Autodesk Inventor part; units mm, degrees
(part 4 of 4)
  line L354 (-31.6525, 241.1962) -> (-31.6525, 254.1962)
  line L355 (-17.6525, 241.1962) -> (-17.6525, 254.1962)
  line L356 (-31.1525, 240.6962) -> (-18.1525, 240.6962)
  line L357 (-31.1525, 254.6962) -> (-18.1525, 254.6962)
  arc A352 (-31.6525, 241.1962) -> (-31.1525, 240.6962) centre (-31.1525, 241.1962) ccw
  arc A353 (-31.1525, 254.6962) -> (-31.6525, 254.1962) centre (-31.1525, 254.1962) ccw
  arc A354 (-18.1525, 240.6962) -> (-17.6525, 241.1962) centre (-18.1525, 241.1962) ccw
  arc A355 (-17.6525, 254.1962) -> (-18.1525, 254.6962) centre (-18.1525, 254.1962) ccw
  line L358 (-31.6525, 265.0087) -> (-31.6525, 278.0087)
  line L359 (-17.6525, 265.0087) -> (-17.6525, 278.0087)
  line L360 (-31.1525, 264.5087) -> (-18.1525, 264.5087)
  line L361 (-31.1525, 278.5087) -> (-18.1525, 278.5087)
  arc A356 (-31.6525, 265.0087) -> (-31.1525, 264.5087) centre (-31.1525, 265.0087) ccw
  arc A357 (-31.1525, 278.5087) -> (-31.6525, 278.0087) centre (-31.1525, 278.0087) ccw
  arc A358 (-18.1525, 264.5087) -> (-17.6525, 265.0087) centre (-18.1525, 265.0087) ccw
  arc A359 (-17.6525, 278.0087) -> (-18.1525, 278.5087) centre (-18.1525, 278.0087) ccw
  line L362 (-31.6525, 288.8212) -> (-31.6525, 301.8212)
  line L363 (-17.6525, 288.8212) -> (-17.6525, 301.8212)
  line L364 (-31.1525, 288.3212) -> (-18.1525, 288.3212)
  line L365 (-31.1525, 302.3212) -> (-18.1525, 302.3212)
  arc A360 (-31.6525, 288.8212) -> (-31.1525, 288.3212) centre (-31.1525, 288.8212) ccw
  arc A361 (-31.1525, 302.3212) -> (-31.6525, 301.8212) centre (-31.1525, 301.8212) ccw
  arc A362 (-18.1525, 288.3212) -> (-17.6525, 288.8212) centre (-18.1525, 288.8212) ccw
  arc A363 (-17.6525, 301.8212) -> (-18.1525, 302.3212) centre (-18.1525, 301.8212) ccw
  line L366 (-31.6525, 315.015) -> (-31.6525, 328.015)
  line L367 (-17.6525, 315.015) -> (-17.6525, 328.015)
  line L368 (-31.1525, 314.515) -> (-18.1525, 314.515)
  line L369 (-31.1525, 328.515) -> (-18.1525, 328.515)
  arc A364 (-31.6525, 315.015) -> (-31.1525, 314.515) centre (-31.1525, 315.015) ccw
  arc A365 (-31.1525, 328.515) -> (-31.6525, 328.015) centre (-31.1525, 328.015) ccw
  arc A366 (-18.1525, 314.515) -> (-17.6525, 315.015) centre (-18.1525, 315.015) ccw
  arc A367 (-17.6525, 328.015) -> (-18.1525, 328.515) centre (-18.1525, 328.015) ccw
  line L370 (-31.6525, 334.065) -> (-31.6525, 347.065)
  line L371 (-17.6525, 334.065) -> (-17.6525, 347.065)
  line L372 (-31.1525, 333.565) -> (-18.1525, 333.565)
  line L373 (-31.1525, 347.565) -> (-18.1525, 347.565)
  arc A368 (-31.6525, 334.065) -> (-31.1525, 333.565) centre (-31.1525, 334.065) ccw
  arc A369 (-31.1525, 347.565) -> (-31.6525, 347.065) centre (-31.1525, 347.065) ccw
  arc A370 (-18.1525, 333.565) -> (-17.6525, 334.065) centre (-18.1525, 334.065) ccw
  arc A371 (-17.6525, 347.065) -> (-18.1525, 347.565) centre (-18.1525, 347.065) ccw
  line L374 (-31.6525, 353.115) -> (-31.6525, 366.115)
  line L375 (-17.6525, 353.115) -> (-17.6525, 366.115)
  line L376 (-31.1525, 352.615) -> (-18.1525, 352.615)
  line L377 (-31.1525, 366.615) -> (-18.1525, 366.615)
  arc A372 (-31.6525, 353.115) -> (-31.1525, 352.615) centre (-31.1525, 353.115) ccw
  arc A373 (-31.1525, 366.615) -> (-31.6525, 366.115) centre (-31.1525, 366.115) ccw
  arc A374 (-18.1525, 352.615) -> (-17.6525, 353.115) centre (-18.1525, 353.115) ccw
  arc A375 (-17.6525, 366.115) -> (-18.1525, 366.615) centre (-18.1525, 366.115) ccw
  line L378 (-15.1275, 21.4775) -> (-15.1275, 369.14)
  line L379 (-134.19, 21.4775) -> (-134.19, 369.14)
  line L380 (-15.1275, 21.4775) -> (-134.19, 21.4775)
  line L381 (-15.1275, 369.14) -> (-134.19, 369.14)
  point P0 (0, 0)
  point P1 (-118.165, 271.6525)
  point P2 (-117.665, 272.1525)
  point P3 (-117.665, 285.1525)
  point P4 (-118.165, 285.6525)
  point P5 (-131.665, 285.1525)
  point P6 (-131.665, 272.1525)
  point P7 (-107.8525, 315.015)
  point P8 (-107.3525, 314.515)
  point P9 (-94.3525, 314.515)
  point P10 (-93.8525, 315.015)
  point P11 (-93.8525, 328.015)
  point P12 (-94.3525, 328.515)
  point P13 (-107.8525, 328.015)
  point P14 (-93.8525, 334.065)
  point P15 (-93.8525, 347.065)
  point P16 (-94.3525, 347.565)
  point P17 (-107.3525, 347.565)
  point P18 (-107.8525, 347.065)
  point P19 (-107.8525, 334.065)
  point P20 (-107.3525, 352.615)
  point P21 (-94.3525, 352.615)
  point P22 (-93.8525, 353.115)
  point P23 (-94.3525, 366.615)
  point P24 (-107.3525, 366.615)
  point P25 (-107.8525, 366.115)
  point P26 (-107.8525, 353.115)
  point P27 (-31.1525, 314.515)
  point P28 (-18.1525, 314.515)
  point P29 (-17.6525, 315.015)
  point P30 (-17.6525, 328.015)
  point P31 (-31.1525, 328.515)
  point P32 (-31.6525, 328.015)
  point P33 (-31.6525, 315.015)
  point P34 (-31.1525, 352.615)
  point P35 (-18.1525, 352.615)
  point P36 (-17.6525, 353.115)
  point P37 (-17.6525, 366.115)
  point P38 (-18.1525, 366.615)
  point P39 (-31.1525, 366.615)
  point P40 (-31.6525, 366.115)
  point P41 (-31.6525, 353.115)
  point P42 (-50.2025, 274.0337)
  point P43 (-37.2025, 274.0337)
  point P44 (-36.7025, 274.5337)
  point P45 (-36.7025, 287.5337)
  point P46 (-37.2025, 288.0337)
  point P47 (-50.2025, 288.0337)
  point P48 (-50.7025, 287.5337)
  point P49 (-50.7025, 274.5337)
  point P50 (-49.2025, 289.4718)
  point P51 (-35.2025, 289.4718)
  point P52 (-34.7025, 289.9717)
  point P53 (-34.7025, 295.9717)
  point P54 (-35.2025, 296.4717)
  point P55 (-49.2025, 296.4717)
  point P56 (-49.7025, 289.9717)
  point P57 (-107.3525, 281.1775)
  point P58 (-94.3525, 281.1775)
  point P59 (-94.3525, 295.1775)
  point P60 (-107.8525, 294.6775)
  point P61 (-107.8525, 281.6775)
  point P62 (-91.8525, 297.1155)
  point P63 (-91.8525, 303.1155)
  point P64 (-92.3525, 303.6155)
  point P65 (-106.3525, 303.6155)
  point P66 (-106.8525, 303.1155)
  point P67 (-106.8525, 297.1155)
  point P68 (-49.2025, 265.5957)
  point P69 (-35.2025, 265.5957)
  point P70 (-34.7025, 266.0958)
  point P71 (-34.7025, 272.0957)
  point P72 (-35.2025, 272.5957)
  point P73 (-49.2025, 272.5957)
  point P74 (-49.7025, 266.0958)
  point P75 (-69.2525, 278.7962)
  point P76 (-56.2525, 278.7962)
  point P77 (-55.7525, 279.2962)
  point P78 (-55.7525, 292.2963)
  point P79 (-56.2525, 292.7963)
  point P80 (-69.2525, 292.7963)
  point P81 (-69.7525, 292.2963)
  point P82 (-69.7525, 279.2962)
  point P83 (-68.2525, 294.2343)
  point P84 (-54.2525, 294.2343)
  point P85 (-53.7525, 294.7342)
  point P86 (-53.7525, 300.7342)
  point P87 (-54.2525, 301.2342)
  point P88 (-68.2525, 301.2342)
  point P89 (-68.7525, 300.7342)
  point P90 (-68.7525, 294.7342)
  point P91 (-88.3025, 314.515)
  point P92 (-75.3025, 314.515)
  point P93 (-74.8025, 315.015)
  point P94 (-74.8025, 328.015)
  point P95 (-75.3025, 328.515)
  point P96 (-88.3025, 328.515)
  point P97 (-88.8025, 328.015)
  point P98 (-88.8025, 315.015)
  point P99 (-118.165, 290.7025)
  point P100 (-117.665, 291.2025)
  point P101 (-117.665, 304.2025)
  point P102 (-118.165, 304.7025)
  point P103 (-131.165, 304.7025)
  point P104 (-131.665, 304.2025)
  point P105 (-131.665, 291.2025)
  point P106 (-31.1525, 288.3212)
  point P107 (-18.1525, 288.3212)
  point P108 (-17.6525, 288.8212)
  point P109 (-17.6525, 301.8212)
  point P110 (-18.1525, 302.3212)
  point P111 (-31.1525, 302.3212)
  point P112 (-31.6525, 301.8212)
  point P113 (-31.6525, 288.8212)
  point P114 (-31.1525, 333.565)
  point P115 (-17.6525, 334.065)
  point P116 (-17.6525, 347.065)
  point P117 (-18.1525, 347.565)
  point P118 (-31.1525, 347.565)
  point P119 (-31.6525, 347.065)
  point P120 (-31.6525, 334.065)
  point P121 (-31.1525, 264.5087)
  point P122 (-18.1525, 264.5087)
  point P123 (-17.6525, 265.0088)
  point P124 (-17.6525, 278.0088)
  point P125 (-18.1525, 278.5087)
  point P126 (-31.1525, 278.5087)
  point P127 (-31.6525, 278.0088)
  point P128 (-31.6525, 265.0088)
  point P129 (-88.3025, 352.615)
  point P130 (-75.3025, 352.615)
  point P131 (-74.8025, 353.115)
  point P132 (-75.3025, 366.615)
  point P133 (-88.3025, 366.615)
  point P134 (-88.8025, 366.115)
  point P135 (-88.8025, 353.115)
  point P136 (-88.3025, 285.94)
  point P137 (-75.3025, 285.94)
  point P138 (-74.8025, 286.44)
  point P139 (-74.8025, 299.44)
  point P140 (-75.3025, 299.94)
  point P141 (-88.3025, 299.94)
  point P142 (-88.8025, 299.44)
  point P143 (-88.8025, 286.44)
  point P144 (-92.3525, 272.7395)
  point P145 (-92.3525, 279.7395)
  point P146 (-106.3525, 279.7395)
  point P147 (-106.8525, 273.2395)
  point P148 (-68.2525, 270.3582)
  point P149 (-54.2525, 270.3582)
  point P150 (-53.7525, 270.8582)
  point P151 (-53.7525, 276.8582)
  point P152 (-54.2525, 277.3582)
  point P153 (-68.7525, 270.8582)
  point P154 (-88.3025, 262.1275)
  point P155 (-75.3025, 262.1275)
  point P156 (-74.8025, 262.6275)
  point P157 (-75.3025, 276.1275)
  point P158 (-88.3025, 276.1275)
  point P159 (-88.8025, 275.6275)
  point P160 (-88.8025, 262.6275)
  point P161 (-50.2025, 333.565)
  point P162 (-36.7025, 334.065)
  point P163 (-36.7025, 347.065)
  point P164 (-37.2025, 347.565)
  point P165 (-50.2025, 347.565)
  point P166 (-50.7025, 347.065)
  point P167 (-50.7025, 334.065)
  point P168 (-88.3025, 333.565)
  point P169 (-75.3025, 333.565)
  point P170 (-74.8025, 334.065)
  point P171 (-74.8025, 347.065)
  point P172 (-75.3025, 347.565)
  point P173 (-88.3025, 347.565)
  point P174 (-88.8025, 347.065)
  point P175 (-88.8025, 334.065)
  point P176 (-50.2025, 200.215)
  point P177 (-37.2025, 200.215)
  point P178 (-36.7025, 200.715)
  point P179 (-36.7025, 213.715)
  point P180 (-37.2025, 214.215)
  point P181 (-50.2025, 214.215)
  point P182 (-50.2025, 238.315)
  point P183 (-37.2025, 238.315)
  point P184 (-36.7025, 238.815)
  point P185 (-36.7025, 251.815)
  point P186 (-37.2025, 252.315)
  point P187 (-50.7025, 251.815)
  point P188 (-50.7025, 238.815)
  point P189 (-131.165, 185.9275)
  point P190 (-118.165, 185.9275)
  point P191 (-117.665, 186.4275)
  point P192 (-117.665, 199.4275)
  point P193 (-131.665, 199.4275)
  point P194 (-131.665, 186.4275)
  point P195 (-131.165, 204.9775)
  point P196 (-118.165, 204.9775)
  point P197 (-117.665, 205.4775)
  point P198 (-118.165, 218.9775)
  point P199 (-131.165, 218.9775)
  dimension "d68" = 10
  dimension "d69" = 10
extrude "Extrusion2" cut sketch "Sketch4" against normal blind 2 contours L2 A1 L5 A3 L3 A2 L4 A0 | L6 A5 L9 A7 L7 A6 L8 A4 | L10 A9 L13 A11 L11 A10 L12 A8 | L14 A13 L17 A15 L15 A14 L16 A12 | L18 A17 L21 A19 L19 A18 L20 A16 | L22 A21 L25 A23 L23 A22 L24 A20 | L26 A25 L29 A27 L27 A26 L28 A24 | L30 A29 L33 A31 L31 A30 L32 A28 | L34 A33 L37 A35 L35 A34 L36 A32 | L38 A37 L41 A39 L39 A38 L40 A36 | L42 A41 L45 A43 L43 A42 L44 A40 | L46 A45 L49 A47 L47 A46 L48 A44 | L50 A49 L53 A51 L51 A50 L52 A48 | L54 A53 L57 A55 L55 A54 L56 A52 | L58 A57 L61 A59 L59 A58 L60 A56 | L62 A61 L65 A63 L63 A62 L64 A60 | L66 A65 L69 A67 L67 A66 L68 A64 | L70 A69 L73 A71 L71 A70 L72 A68 | L74 A73 L77 A75 L75 A74 L76 A72 | L78 A77 L81 A79 L79 A78 L80 A76 | L82 A81 L85 A83 L83 A82 L84 A80 | L86 A85 L89 A87 L87 A86 L88 A84 | L90 A89 L93 A91 L91 A90 L92 A88 | L94 A93 L97 A95 L95 A94 L96 A92 | L98 A97 L101 A99 L99 A98 L100 A96 | L102 A101 L105 A103 L103 A102 L104 A100 | L106 A105 L109 A107 L107 A106 L108 A104 | L110 A109 L113 A111 L111 A110 L112 A108 | L114 A113 L117 A115 L115 A114 L116 A112 | L118 A117 L121 A119 L119 A118 L120 A116 | L122 A121 L125 A123 L123 A122 L124 A120 | L126 A125 L129 A127 L127 A126 L128 A124 | L130 A129 L133 A131 L131 A130 L132 A128 | L134 A133 L137 A135 L135 A134 L136 A132 | L138 A137 L141 A139 L139 A138 L140 A136 | L142 A141 L145 A143 L143 A142 L144 A140 | L146 A145 L149 A147 L147 A146 L148 A144 | L150 A149 L153 A151 L151 A150 L152 A148 | L154 A153 L157 A155 L155 A154 L156 A152 | L158 A157 L161 A159 L159 A158 L160 A156 | L162 A161 L165 A163 L163 A162 L164 A160 | L166 A165 L169 A167 L167 A166 L168 A164 | L170 A169 L173 A171 L171 A170 L172 A168 | L174 A173 L177 A175 L175 A174 L176 A172 | L178 A177 L181 A179 L179 A178 L180 A176 | L182 A181 L185 A183 L183 A182 L184 A180 | L186 A185 L189 A187 L187 A186 L188 A184 | L190 A189 L193 A191 L191 A190 L192 A188 | L194 A193 L197 A195 L195 A194 L196 A192 | L198 A197 L201 A199 L199 A198 L200 A196 | L202 A201 L205 A203 L203 A202 L204 A200 | L206 A205 L209 A207 L207 A206 L208 A204 | L210 A209 L213 A211 L211 A210 L212 A208 | L214 A213 L217 A215 L215 A214 L216 A212 | L218 A217 L221 A219 L219 A218 L220 A216 | L222 A221 L225 A223 L223 A222 L224 A220 | L226 A225 L229 A227 L227 A226 L228 A224 | L230 A229 L233 A231 L231 A230 L232 A228 | L234 A233 L237 A235 L235 A234 L236 A232 | L238 A237 L241 A239 L239 A238 L240 A236 | L242 A241 L245 A243 L243 A242 L244 A240 | L246 A245 L249 A247 L247 A246 L248 A244 | L250 A249 L253 A251 L251 A250 L252 A248 | L254 A253 L257 A255 L255 A254 L256 A252 | L258 A257 L261 A259 L259 A258 L260 A256 | L262 A261 L265 A263 L263 A262 L264 A260 | L266 A265 L269 A267 L267 A266 L268 A264 | L270 A269 L273 A271 L271 A270 L272 A268 | L274 A273 L277 A275 L275 A274 L276 A272 | L278 A277 L281 A279 L279 A278 L280 A276 | L282 A281 L285 A283 L283 A282 L284 A280 | L286 A285 L289 A287 L287 A286 L288 A284 | L290 A289 L293 A291 L291 A290 L292 A288 | L294 A293 L297 A295 L295 A294 L296 A292 | L298 A297 L301 A299 L299 A298 L300 A296 | L302 A301 L305 A303 L303 A302 L304 A300 | L306 A305 L309 A307 L307 A306 L308 A304 | L310 A309 L313 A311 L311 A310 L312 A308 | L314 A313 L317 A315 L315 A314 L316 A312 | L318 A317 L321 A319 L319 A318 L320 A316 | L322 A321 L325 A323 L323 A322 L324 A320 | L326 A325 L329 A327 L327 A326 L328 A324 | L330 A329 L333 A331 L331 A330 L332 A328 | L334 A333 L337 A335 L335 A334 L336 A332 | L338 A337 L341 A339 L339 A338 L340 A336 | L342 A341 L345 A343 L343 A342 L344 A340 | L346 A345 L349 A347 L347 A346 L348 A344 | L350 A349 L353 A351 L351 A350 L352 A348 | L354 A353 L357 A355 L355 A354 L356 A352 | L358 A357 L361 A359 L359 A358 L360 A356 | L362 A361 L365 A363 L363 A362 L364 A360 | L366 A365 L369 A367 L367 A366 L368 A364 | L370 A369 L373 A371 L371 A370 L372 A368 | L374 A373 L377 A375 L375 A374 L376 A372
body "Solid1"
